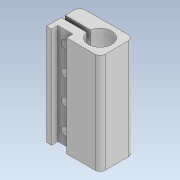
# Autodesk Inventor part: ADAPTATEUR
Saved by Autodesk Inventor 2020 (Build 240168000, 168)
## iProperties
Created: 2020-07-01
Part Number: ADAPTATEUR
Material: Generic
Document SubType Name: Modeling
Designer: Admin
Density: 1 g/cm^3
Appearance: Default
Author: Admin
Autodesk Inventor part; units mm, degrees
ref_plane "YZ Plane" through (0, 0, 0) normal (1, 0, 0) x (0, 1, 0)
ref_plane "XZ Plane" through (0, 0, 0) normal (0, 1, 0) x (-1, 0, 0)
ref_plane "XY Plane" through (0, 0, 0) normal (0, 0, 1) x (1, 0, 0)
sketch "Sketch1" plane through (0, 0, 0) normal (0, 1, 0) x (-1, 0, 0)
  line L0 (0, 0) -> (21.3, 0)
  line L1 (21.3, 0) -> (21.3, -13.3)
  line L2 (21.3, -13.3) -> (0, -13.3)
  line L3 (0, -13.3) -> (0, 0)
  dimension "d0" = 21.3
  dimension "d1" = 13.3
  constraints: 8 end point, 2 parallel, 1 horizontal, 1 perpendicular
  measures "d0" distance of L1.end L2.end
  measures "d1" distance of L2.end L0.start
extrude "Extrusion1" add sketch "Sketch1" along normal blind 40
sketch "Sketch2" plane through (0, 40, 0) normal (0, 1, 0) x (1, 0, 0)
  circle A0 centre (-6.65, 6.65) radius 4.65
  line L0 (0, 0) -> (0, 13.3) projected
  line L1 (-21.3, 0) -> (0, 0) projected
  dimension "d4" = 9.3
  dimension "d5" = 6.65
  dimension "d6" = 6.65
  constraints: 1 centre point
  measures "d4" diameter of A0
  measures "d5" distance from line of L0 A0.centre
  measures "d6" distance from line of L1 A0.centre
extrude "Extrusion2" cut sketch "Sketch2" against normal through all
sketch "Sketch3" plane through (0, 40, 0) normal (0, 1, 0) x (1, 0, 0)
  line L0 (-21.3, 5.9) -> (-9.3, 5.9)
  line L1 (-9.3, 5.9) -> (-9.3, 7.4)
  line L2 (-9.3, 7.4) -> (-21.3, 7.4)
  line L3 (-21.3, 7.4) -> (-21.3, 5.9)
  line L4 (0, 13.3) -> (-21.3, 13.3) projected
  line L5 (-21.3, 13.3) -> (-21.3, 0) projected
  point P0 (0, 0)
  dimension "d9" = 1.5
  dimension "d10" = 5.9
  dimension "d11" = 12
  constraints: 8 end point, 2 parallel, 1 horizontal, 1 perpendicular, 1 point on line
  measures "d9" distance of L0.end L1.end
  measures "d10" distance between parallel lines of L4 L2
  measures "d11" distance of L1.end L2.end
extrude "Extrusion3" cut sketch "Sketch3" against normal through all
sketch "Sketch4" plane through (0, 40, 0) normal (0, 1, 0) x (1, 0, 0)
  line L0 (-19.3, 0) -> (-13.3, 0)
  line L1 (-13.3, 0) -> (-13.3, 2.5)
  line L2 (-13.3, 2.5) -> (-19.3, 2.5)
  line L3 (-19.3, 2.5) -> (-19.3, 0)
  line L4 (-21.3, 5.9) -> (-21.3, 0) projected
  line L5 (-21.3, 0) -> (0, 0) projected
  dimension "d14" = 2.5
  dimension "d15" = 6
  dimension "d16" = 2
  constraints: 8 end point, 2 parallel, 1 horizontal, 1 perpendicular, 1 point on line
  measures "d14" distance of L2.end L0.start
  measures "d15" distance of L1.end L2.end
  measures "d16" distance between parallel lines of L3 L4
extrude "Extrusion4" cut sketch "Sketch4" against normal through all
sketch "Sketch5" plane through (0, 0, -13.3) normal (0, 0, -1) x (-1, 0, 0)
  circle A0 centre (16.3, 35) radius 1.6
  line L0 (21.3, 0) -> (21.3, 40) projected
  line L1 (0, 40) -> (21.3, 40) projected
  point P0 (0, 0)
  dimension "d19" = 3.2
  dimension "d20" = 5
  dimension "d21" = 5
  constraints: 1 centre point
  measures "d19" diameter of A0
  measures "d20" distance from line of L0 A0.centre
  measures "d21" distance from line of A0.centre L1
extrude "Extrusion5" cut sketch "Sketch5" against normal through all
pattern_linear "Rectangular Pattern1" count 4 spacing 10 along (0, -1, 0) of "Extrusion5"
sketch "Sketch6" plane through (0, 0, -13.3) normal (0, 0, -1) x (-1, 0, 0)
  line L0 (11.2391, 0) -> (11.2391, 40) projected
  circle A0 centre (16.3, 35) radius 3
  line L1 (21.3, 0) -> (21.3, 40) projected
  line L2 (0, 40) -> (21.3, 40) projected
  point P0 (0, 0)
  dimension "d27" = 6
  dimension "d28" = 5
  dimension "d29" = 5
  constraints: 1 centre point
  measures "d27" diameter of A0
  measures "d28" distance from line of L1 A0.centre
  measures "d29" distance from line of L2 A0.centre
extrude "Extrusion6" cut sketch "Sketch6" against normal blind 3
pattern_linear "Rectangular Pattern2" count 4 spacing 10 along (0, -1, 0) of "Extrusion6"
fillet "Fillet1" radius 2 3 edges at (0, 20, -13.3) (-21.3, 20, -13.3) (0, 20, 0)
equation "\"d6\" = d5"
body "Solid1"
